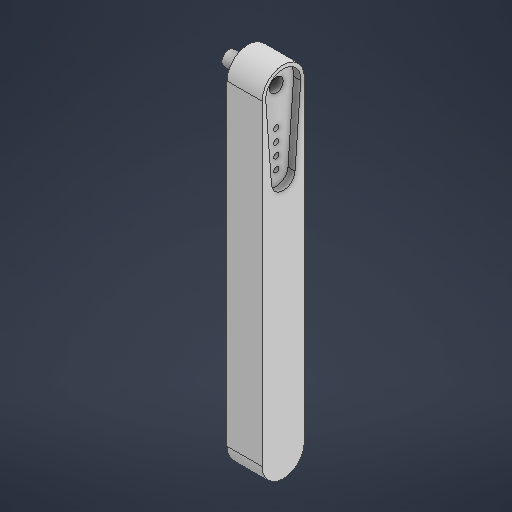
# Autodesk Inventor part: Payload Release Actuator Arm
Saved by Autodesk Inventor 2026.1 (Build 301233000, 233)
## iProperties
Created: 2026-03-29
Part Number: Payload Release Actuator Arm
Material: Generic
Document SubType Name: Modeling
Designer: elisa
Density: 1 g/cm^3
Appearance: Default
Author: elisa
Autodesk Inventor part; units mm, degrees
ref_plane "YZ Plane" through (0, 0, 0) normal (1, 0, 0) x (0, 1, 0)
ref_plane "XZ Plane" through (0, 0, 0) normal (0, 1, 0) x (-1, 0, 0)
ref_plane "XY Plane" through (0, 0, 0) normal (0, 0, 1) x (1, 0, 0)
sketch "Sketch1" plane through (0, 0, 0) normal (1, 0, 0) x (0, 1, 0)
  arc A0 (0, -6) -> (0, 6) centre (0, 0) ccw
  line L0 (0, 6) -> (-90, 6)
  line L1 (-90, -6) -> (0, -6)
  arc A1 (-90, 6) -> (-90, -6) centre (-90, 0) ccw
  line L2 (0, 101) -> (0, 6) construction
  line L3 (0, -6) -> (0, -101) construction
  dimension "d1" = 12
  dimension "d3" = 90
  constraints: 8 end point, 4 point on circle, 2 centre point, 2 parallel, 2 vertical, 1 coincident, 1 equal radius, 1 horizontal
  measures "d1" diameter of A0
  measures "d3" distance of L1.start L1.end
extrude "Main Arm" add sketch "Sketch1" along normal blind 10
sketch "Sketch2" plane through (10, 0, 0) normal (1, 0, 0) x (0, 0, -1)
  arc A0 (4.9681, -0.3712) -> (-4.9681, -0.3712) centre (0, 0) ccw
  arc A1 (-3.3596, -21.897) -> (3.3596, -21.897) centre (0, -21.646) ccw
  line L0 (-4.9681, -0.3712) -> (-3.3596, -21.897)
  line L1 (4.9681, -0.3712) -> (3.3596, -21.897)
  point P0 (6, 0)
  dimension "d11" = 9.964
  dimension "d12" = 6.738
  dimension "d13" = 21.646
  constraints: 4 end point, 4 point on circle, 4 tangent, 2 centre point, 1 other
  measures "d11" diameter of A0
  measures "d12" diameter of A1
  measures "d13" distance of A1.centre A0.centre
extrude "Extrusion2" cut sketch "Sketch2" against normal blind 2
sketch "Sketch3" plane through (8, 0, 0) normal (1, 0, 0) x (0, 0, -1)
  circle A0 centre (0, -10.588) radius 0.75
  line L0 (0, 125) -> (0, -125) construction
  circle A1 centre (0, -14.021) radius 0.75
  circle A2 centre (0, -17.454) radius 0.75
  circle A3 centre (0, -20.887) radius 0.75
  point P0 (0, 0)
  dimension "d14" = 1.5
  dimension "d15" = 10.588
  dimension "d19" = 3.433
  constraints: 4 centre point, 2 end point, 2 vertical, 1 midpoint, 6 other
  measures "d14" diameter of A0
  measures "d15" distance of A0.centre point (0, 0)
  measures "d19" distance of A0.centre A1.centre
extrude "Extrusion3" cut sketch "Sketch3" against normal blind 5
sketch "Sketch4" plane through (8, 0, 0) normal (1, 0, 0) x (0, 0, -1)
  circle A0 centre (0, 0) radius 2
  dimension "d26" = 4
  constraints: 1 centre point, 1 coincident
  measures "d26" diameter of A0
extrude "Extrusion4" cut sketch "Sketch4" against normal blind 5.5
sketch "Sketch5" plane through (0, 0, 0) normal (-1, 0, 0) x (0, 0, 1)
  circle A0 centre (0, 0) radius 2 projected
  circle A1 centre (0, 0) radius 2.25
  dimension "d29" = 4.5
  constraints: 1 centre point, 1 coincident
  measures "d29" diameter of A1
extrude "Extrusion5" add sketch "Sketch5" along normal blind 5.5 contours A0
body "Solid1"
